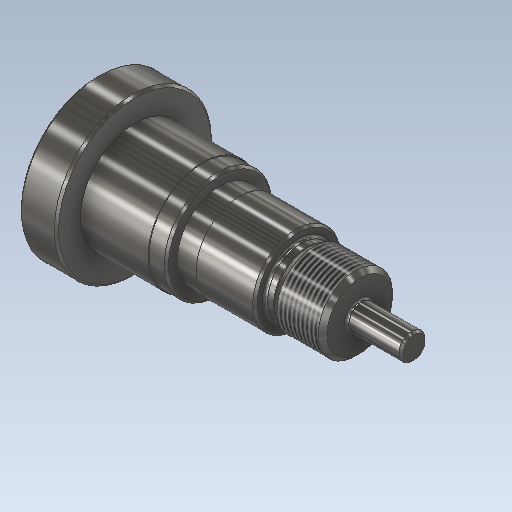
# Autodesk Inventor part: Shoulder_Shaft_Pitch
Saved by Autodesk Inventor 2021.4 (Build 254397000, 397)
## iProperties
Created: 2020-04-22
Part Number: Shoulder_Shaft_Pitch
Material: Stahl, hochfest, niedrig legiert
Document SubType Name: Modeling
Designer: Alex
Density: 7.85 g/cm^3
Appearance: Stahl - poliert
Mass: 207.174 g
Surface Area: 69.5444 cm^2
Volume: 26.3916 cm^3
Author: Alex
Autodesk Inventor part; units mm, degrees
ref_plane "YZ Plane" through (0, 0, 0) normal (1, 0, 0) x (0, 1, 0)
ref_plane "XZ Plane" through (0, 0, 0) normal (0, 1, 0) x (-1, 0, 0)
ref_plane "XY Plane" through (0, 0, 0) normal (0, 0, 1) x (1, 0, 0)
sketch "Skizze1" plane through (0, 0, 0) normal (0, 0, 1) x (1, 0, 0)
  line L0 (0, 0) -> (0, 18)
  line L1 (8.5, 12.5) -> (24, 12.5)
  line L2 (46, 10) -> (46, 8.3)
  arc A0 (46, 8.3) -> (46.6, 7.7) centre (46.6, 8.3) ccw
  line L3 (46.6, 7.7) -> (47.9536, 7.7)
  arc A1 (47.9536, 7.7) -> (48.2536, 7.7804) centre (47.9536, 8.3) ccw
  line L4 (48.2536, 7.7804) -> (49.5, 8.5)
  line L5 (72.5, 3) -> (72.5, 0)
  line L6 (0, 0) -> (72.5, 0)
  line L7 (-14.5, 0) -> (87, 0) construction
  line L8 (32.5, 10) -> (46, 10)
  line L9 (60, 7.5) -> (60, 3)
  line L10 (60, 3) -> (72.5, 3)
  line L11 (49.5, 8.5) -> (59, 8.5)
  line L12 (60, 7.5) -> (59, 8.5)
  line L13 (64, -11.5) -> (64, 11.5) construction
  line L14 (0, 18) -> (8.5, 18)
  line L15 (8.5, 18) -> (8.5, 12.5)
  line L16 (24, 12.5) -> (24, 12.3)
  line L17 (32.5, 10) -> (32.5, 9.8)
  line L18 (32.5, 9.8) -> (28, 9.8)
  line L19 (28, 9.8) -> (28, 12.3)
  line L20 (28, 12.3) -> (24, 12.3)
  point P0 (60, 8.5)
  dimension "d0" = 25
  dimension "d3" = 0.6
  dimension "d4" = 0.6
  dimension "d7" = 3.5
  dimension "d35" = 15.4
  dimension "d36" = 24
  dimension "d37" = 32.5
  dimension "d38" = 20
  dimension "d39" = 46
  dimension "d40" = 17
  dimension "d41" = 30
  dimension "d42" = 1
  dimension "d43" = 1
  dimension "d44" = 60
  dimension "d45" = 6
  dimension "d56" = 8.5
  dimension "d57" = 36
  dimension "d58" = 8.5
  dimension "d60" = 0.2
  dimension "d61" = 0.2
  dimension "d62" = 4
  constraints: 38 end point, 6 horizontal, 6 perpendicular, 4 point on circle, 4 tangent, 4 vertical, 2 centre point, 2 point on line
  measures "d0" diameter of L1 L6
  measures "d3" radius of A0
  measures "d4" radius of A1
  measures "d7" distance from line of L4.end L2
  measures "d35" diameter of L3 L6
  measures "d36" distance from line of L1.end L0
  measures "d37" distance from line of L8.start L0
  measures "d38" diameter of L8 L6
  measures "d39" distance between parallel lines of L2 L0
  measures "d40" diameter of L11 L7
  measures "d41" angle of L11 L4
  measures "d42" distance of L9.start point (60, 8.5)
  measures "d43" distance of L11.end point (60, 8.5)
  measures "d44" distance from line of point (60, 8.5) L0
  measures "d45" diameter of L10 L7
  measures "d56" distance between parallel lines of L5 L13
  measures "d57" diameter of L14 L7
  measures "d58" distance between parallel lines of L0 L15
  measures "d60" distance between parallel lines of L8 L18
  measures "d61" distance between parallel lines of L20 L1
  measures "d62" distance from line of L19 L1.end
revolve "Grundprofil" add sketch "Skizze1" angle 360 about axis through (-10, 0, 0) along (1, 0, 0)
sketch "Skizze2" plane through (0, 0, 0) normal (-1, 0, 0) x (0, 0, 1)
  point P0 (0, 0)
  point P1 (0, 0)
  constraints: 1 coincident
hole "M8 Sacklochbohrung" at (0, 0, 0) direction (1, 0, 0) diameter 6.647 depth 20 tip angle 118 thread size "M8x1.25" class "6H" standard "ISO Metric profile"
thread "M17x1mm Aussenfeingewinde" size "M17x1" class "6g" standard "ISO Metric profile" full length
fillet "Kerbwirkungsreduktion 0.5mm" radius 0.5 1 edges at (60, -3, 0)
chamfer "Fase4" distance 0.5 angle 45 5 edges at (0, -18, 0) (8.5, -18, 0) (28, -12.3, 0) (46, -10, 0) (72.5, -3, 0)
equation "\"d43\" = d42"
